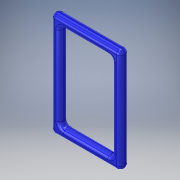
# Autodesk Inventor part: winding
Saved by Autodesk Inventor 2019.4 (Build 234330000, 330)
## iProperties
Created: 2019-10-01
Part Number: winding
Material: Generic
Document SubType Name: Modeling
Designer: cdi
Density: 1 g/cm^3
Appearance: Blue - Wall Paint - Glossy
Author: cdi
Autodesk Inventor part; units mm, degrees
ref_plane "YZ Plane" through (0, 0, 0) normal (1, 0, 0) x (0, 1, 0)
ref_plane "XZ Plane" through (0, 0, 0) normal (0, 1, 0) x (-1, 0, 0)
ref_plane "XY Plane" through (0, 0, 0) normal (0, 0, 1) x (1, 0, 0)
sketch "Sketch1" plane through (0, 0, 0) normal (0, 0, 1) x (1, 0, 0)
  line L0 (-3, -5) -> (-3, 5)
  line L1 (-3, 5) -> (3, 5)
  line L2 (3, 5) -> (3, -5)
  line L3 (3, -5) -> (-3, -5)
  line L4 (-3, -5) -> (3, 5) construction
  line L5 (-3, 5) -> (3, -5) construction
  line L6 (4, 6) -> (-4, 6)
  line L7 (-4, 6) -> (-4, -6)
  line L8 (-4, -6) -> (4, -6)
  line L9 (4, -6) -> (4, 6)
  point P0 (0, 0)
  dimension "d0" = 6
  dimension "d1" = 10
  dimension "d2" = 1
  constraints: 20 end point, 4 parallel, 2 midpoint, 2 perpendicular, 1 vertical, 3 other
  measures "d0" distance of L0.end L1.end
  measures "d1" distance of L1.end L2.end
  measures "d2" distance between parallel lines of L2 L9
extrude "Extrusion1" add sketch "Sketch1" along normal blind 1
fillet "Fillet1" radius 0.45 24 edges at (0, 5, 1) (-3, 0, 1) (-3, 0, 0) (0, -5, 1) (0, -5, 0) (3, 0, 1) (3, 0, 0) (0, 5, 0) (-3, 5, 0.5) (-3, -5, 0.5) (3, -5, 0.5) (3, 5, 0.5) (4, 6, 0.5) (0, 6, 0) (-4, 0, 0) (4, 0, 0) (4, 0, 1) (0, -6, 0) (4, -6, 0.5) (0, -6, 1) (-4, -6, 0.5) (-4, 0, 1) (-4, 6, 0.5) (0, 6, 1)
body "Solid1"
